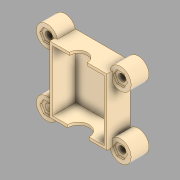
# Autodesk Inventor part: uchwyt_maly_silnik
Saved by Autodesk Inventor 2021 (Build 250183000, 183)
## iProperties
Created: 2022-05-16
Part Number: uchwyt_maly_silnik
Material: PC/ABS Plastic
Document SubType Name: Modeling
Designer: agnpi
Density: 0.357273 g/cm^3
Appearance: Smooth - Off-White
Author: agnpi
Autodesk Inventor part; units mm, degrees
ref_plane "YZ Plane" through (0, 0, 0) normal (1, 0, 0) x (0, 1, 0)
ref_plane "XZ Plane" through (0, 0, 0) normal (0, 1, 0) x (-1, 0, 0)
ref_plane "XY Plane" through (0, 0, 0) normal (0, 0, 1) x (1, 0, 0)
sketch "Sketch1" plane through (0, 0, 0) normal (0, 0, 1) x (1, 0, 0)
  line L0 (-37.1, 0) -> (37.1, 0) projected
  line L1 (0, -33.4) -> (0, 32.4) projected
  line L2 (-14.5, 17) -> (14.5, 17)
  line L3 (14.5, 17) -> (14.5, -17)
  line L4 (14.5, -17) -> (-14.5, -17)
  line L5 (-14.5, -17) -> (-14.5, 17)
  line L6 (-14.5, 17) -> (14.5, -17) construction
  line L7 (14.5, 17) -> (-14.5, -17) construction
  line L8 (-16, 18.5) -> (16, 18.5)
  line L9 (16, 18.5) -> (16, -18.5)
  line L10 (16, -18.5) -> (-16, -18.5)
  line L11 (-16, -18.5) -> (-16, 18.5)
  line L12 (-16, 18.5) -> (16, -18.5) construction
  line L13 (16, 18.5) -> (-16, -18.5) construction
  circle A0 centre (20.5, 17) radius 6
  circle A1 centre (20.5, -18) radius 6
  line L14 (22.5207, 13.5) -> (18.4793, 13.5)
  line L15 (18.4793, 13.5) -> (16.4585, 17)
  line L16 (16.4585, 17) -> (18.4793, 20.5)
  line L17 (18.4793, 20.5) -> (22.5207, 20.5)
  line L18 (22.5207, 20.5) -> (24.5415, 17)
  line L19 (24.5415, 17) -> (22.5207, 13.5)
  line L20 (22.5207, -21.5) -> (18.4793, -21.5)
  line L21 (18.4793, -21.5) -> (16.4585, -18)
  line L22 (16.4585, -18) -> (18.4793, -14.5)
  line L23 (18.4793, -14.5) -> (22.5207, -14.5)
  line L24 (22.5207, -14.5) -> (24.5415, -18)
  line L25 (24.5415, -18) -> (22.5207, -21.5)
  circle A2 centre (-20.5, -18) radius 6
  circle A3 centre (-20.5, 17) radius 6
  point P0 (0, 0)
  point P1 (-16, -14.0314)
  point P2 (-14.5209, -18.5)
  point P3 (-14.6905, 18.5)
  point P4 (-16, 13.0314)
  dimension "d45" = 6
  dimension "d0" = 29
  dimension "d1" = 34
  dimension "d2" = 32
  dimension "d3" = 37
  dimension "d13" = 12
  dimension "d14" = 12
  dimension "d15" = 47
  dimension "d16" = 0
  dimension "d18" = 7
  dimension "d19" = 7
  constraints: 48 end point, 6 parallel, 4 centre point, 4 midpoint, 2 coincident, 2 horizontal, 2 perpendicular, 2 symmetric about line, 2 tangent, 28 other
  measures "d0" distance of L3.end L4.end
  measures "d1" distance of L2.end L3.end
  measures "d2" distance of L9.end L10.end
  measures "d3" distance of L8.end L9.end
  measures "d13" diameter of A0
  measures "d14" diameter of A1
  measures "d16" distance from line of L2 A0.centre
  measures "d18" distance between parallel lines of L14 L17
  measures "d19" distance between parallel lines of L20 L23
extrude "Extrusion1" add sketch "Sketch1" along normal blind 13 contours L11 A3 L5 L0 | L0 L5 L4 L1 L10 A2 L11 | A2 L10 L11 | L11 L8 A3 | A3 L8 L1 L2 | L3 A0 L9 L0 | L0 L9 A1 L10 L1 L4 L3 | L1 L8 A0 L2 | A0 L8 L9 | A1 L9 L10 picked at (-15.7277, -15.917) picked at (-15.7277, 15.2503) picked at (15.7277, 15.2503) picked at (15.7655, -15.848)
extrude "Extrusion2" add sketch "Sketch1" along normal blind 10 contours A0 L8 L9 | A0 L9 L8 | L14 L15 L16 L17 L18 L19
sketch "Sketch3" plane through (-16, -18.5, 13) normal (0, -1, 0) x (1, 0, 0)
  line L0 (32, 0) -> (0, 0) projected
  arc A0 (10, 0) -> (22, 0) centre (16, 0) ccw
  point P0 (16, -13)
  dimension "d36" = 6
  constraints: 2 point on circle, 1 centre point, 1 midpoint, 1 point on line
  measures "d36" radius of A0
extrude "Extrusion6" cut sketch "Sketch3" against normal up to surface (1.5 mm away)
sketch "Sketch4" plane through (-16, 18.5, 13) normal (0, 1, 0) x (1, 0, 0)
  arc A0 (22, 0) -> (10, 0) centre (16, 0) ccw projected
  line L0 (1.5, 0) -> (30.5, 0) projected
  arc A1 (21, 0) -> (11, 0) centre (16, 0) ccw
  point P0 (16, 13)
  point P1 (11, 0)
  dimension "d39" = 5
  constraints: 2 point on circle, 1 centre point, 1 coincident, 1 point on line
  measures "d39" radius of A1
extrude "Extrusion7" cut sketch "Sketch4" against normal up to surface (1.5 mm away) contours L0 A1
extrude "Extrusion8" add sketch "Sketch1" against normal blind 0.01 contours L5 L2 L1 L0 | L0 L1 L4 L5 | L1 L2 L3 L0 | L0 L3 L4 L1
hole "Hole2" at (20.5, 17, 0) direction (0, 0, 1) diameter 4 end through all
extrude "Extrusion10" add sketch "Sketch1" along normal blind 10 contours L11 L10 A2 picked at (-22.9633, -17.9533)
sketch "Sketch6" plane through (0, 0, 13) normal (0, 0, 1) x (1, 0, 0)
  line L0 (22.5377, 13.5) -> (18.4962, 13.5)
  line L1 (18.4962, 13.5) -> (16.4755, 17)
  line L2 (16.4755, 17) -> (18.4962, 20.5)
  line L3 (18.4962, 20.5) -> (22.5377, 20.5)
  line L4 (22.5377, 20.5) -> (24.5584, 17)
  line L5 (24.5584, 17) -> (22.5377, 13.5)
  line L6 (5, 17) -> (14.5, 17) projected
  point P0 (0, 0)
  point P1 (20.5169, 17)
  dimension "d56" = 7
  constraints: 12 end point, 1 parallel, 13 other
  measures "d56" distance between parallel lines of L0 L3
extrude "Extrusion11" cut sketch "Sketch6" against normal blind 4
extrude "Extrusion12" add sketch "Sketch1" along normal blind 10 contours A1 L9 L10 | L10 L9 A1 | L20 L21 L22 L23 L24 L25
hole "Hole3" at (20.5, -18, 0) direction (0, 0, 1) diameter 4 end through all
hole "Hole4" at (-20.5, -18, 0) direction (0, 0, 1) diameter 4 end through all
sketch "Sketch7" plane through (0, 0, 13) normal (0, 0, 1) x (1, 0, 0)
  line L0 (-18.4821, -21.5) -> (-22.5236, -21.5)
  line L1 (-22.5236, -21.5) -> (-23.5436, -19.7333)
  line L2 (-24.5443, -18) -> (-22.5236, -14.5)
  line L3 (-22.5236, -14.5) -> (-18.4821, -14.5)
  line L4 (-18.4821, -14.5) -> (-16.4614, -18)
  line L5 (-16.4614, -18) -> (-18.4821, -21.5)
  line L6 (-16, -18.5) -> (-6, -18.5) projected
  line L7 (-14.5, 17) -> (-5, 17) projected
  line L8 (-23.5436, -19.7333) -> (-24.5443, -18)
  point P0 (0, 0)
  point P1 (-20.5029, -18)
  point P2 (-14.5, -18)
  dimension "d75" = 7
  dimension "d78" = 31.5
  constraints: 14 end point, 1 horizontal, 14 other
  measures "d75" distance between parallel lines of L0 L3
  measures "d78" distance between parallel lines of L7 L3
extrude "Extrusion13" add sketch "Sketch1" along normal blind 10 contours A3 L8 L11 picked at (-22.7049, 16.071)
sketch "Sketch8" plane through (0, 0, 13) normal (0, 0, 1) x (1, 0, 0)
  point P0 (0, 0)
hole "Hole5" at (-20.5, 17, 0) direction (0, 0, 1) diameter 4 end through all
sketch "Sketch9" plane through (0, 0, 13) normal (0, 0, 1) x (1, 0, 0)
  line L0 (-18.4799, 13.5) -> (-22.5213, 13.5)
  line L1 (-22.5213, 13.5) -> (-24.5421, 17)
  line L2 (-24.5421, 17) -> (-22.5213, 20.5)
  line L3 (-22.5213, 20.5) -> (-18.4799, 20.5)
  line L4 (-18.4799, 20.5) -> (-16.4592, 17)
  line L5 (-16.4592, 17) -> (-18.4799, 13.5)
  line L6 (-14.5, 17) -> (-5, 17) projected
  point P0 (0, 0)
  point P1 (-20.5006, 17)
  dimension "d89" = 7
  constraints: 12 end point, 1 point on line, 9 other
  measures "d89" distance between parallel lines of L0 L3
extrude "Extrusion14" cut sketch "Sketch9" against normal blind 4
extrude "Extrusion15" cut sketch "Sketch7" against normal blind 4
sketch "Sketch10" plane through (0, 0, 13) normal (0, 0, 1) x (1, 0, 0)
  line L0 (22.5207, -21.4318) -> (18.4793, -21.4318)
  line L1 (18.4793, -21.4318) -> (16.4585, -17.9318)
  line L2 (16.4585, -17.9318) -> (18.4793, -14.4318)
  line L3 (18.4793, -14.4318) -> (22.5207, -14.4318)
  line L4 (22.5207, -14.4318) -> (24.5415, -17.9318)
  line L5 (24.5415, -17.9318) -> (22.5207, -21.4318)
  line L6 (6, -18.5) -> (-6, -18.5) projected
  arc A0 (16, 13.0314) -> (14.6905, 18.5) centre (20.5, 17) ccw projected
  point P0 (0, 0)
  point P1 (20.5, -17.9318)
  point P2 (14.5, -18)
  point P3 (15.5, 13.6834)
  point P4 (14.5839, 18)
  point P5 (15.6266, 13.5)
  point P6 (15.6266, 20.5)
  dimension "d95" = 7
  dimension "d96" = 34.9318
  dimension "d97" = 13.9659
  constraints: 12 end point, 1 horizontal, 14 other
  measures "d95" distance between parallel lines of L0 L3
  measures "d96" distance of A0.centre point (20.5, -17.932)
  measures "d97" distance from line of A0.centre L4
extrude "Extrusion16" cut sketch "Sketch10" against normal blind 4
sketch "Sketch14" plane through (0, -18.5, 13) normal (0, -1, 0) x (1, 0, 0)
  circle A0 centre (0, -9) radius 2
  line L0 (-14.5209, -13) -> (14.5209, -13) projected
  point P0 (0, -13)
  dimension "d106" = 4
  dimension "d107" = 4
  constraints: 1 centre point
  measures "d106" diameter of A0
  measures "d107" distance from line of L0 A0.centre
extrude "Extrusion18" cut sketch "Sketch14" against normal blind 1
body "Solid1"
